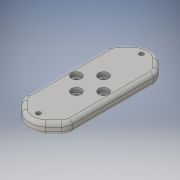
# Autodesk Inventor part: ROV Motor plate
Saved by Autodesk Inventor 2016 (Build 200138000, 138)
## iProperties
Created: 2017-03-09
Part Number: ROV Motor plate
Material: Generic
Document SubType Name: Modeling
Designer: Student
Density: 1 g/cm^3
Appearance: Default
Author: Student
Autodesk Inventor part; units mm, degrees
ref_plane "YZ Plane" through (0, 0, 0) normal (1, 0, 0) x (0, 1, 0)
ref_plane "XZ Plane" through (0, 0, 0) normal (0, 1, 0) x (-1, 0, 0)
ref_plane "XY Plane" through (0, 0, 0) normal (0, 0, 1) x (1, 0, 0)
sketch "Sketch1" plane through (0, 0, 0) normal (0, 1, 0) x (-1, 0, 0)
  line L0 (0, 0) -> (-31.75, 0)
  line L1 (-31.75, 0) -> (-31.75, -77.47)
  line L2 (-31.75, -77.47) -> (0, -77.47)
  line L3 (0, -77.47) -> (0, 0)
  dimension "d0" = 31.75
  dimension "d1" = 77.47
  constraints: 8 end point, 2 parallel, 1 horizontal, 1 perpendicular
  measures "d0" distance of L2.end L1.end
  measures "d1" distance of L1.end L0.end
extrude "Extrusion1" add sketch "Sketch1" along normal blind 7.62
sketch "Sketch2" plane through (0, 7.62, 0) normal (0, 1, 0) x (1, 0, 0)
  line L0 (31.75, 77.47) -> (0, 77.47) projected
  line L1 (0, 0) -> (31.75, 0) projected
  line L2 (0, 77.47) -> (0, 0) projected
  line L3 (31.75, 0) -> (31.75, 77.47) projected
  point P0 (15.875, 74.295)
  point P1 (15.875, 3.175)
  dimension "d6" = 3.175
  dimension "d8" = 15.875
  dimension "d10" = 15.875
  dimension "d37" = 3.175
  measures "d6" distance from line of L1 point (15.875, 3.175)
  measures "d8" distance from line of L2 point (15.875, 3.175)
  measures "d10" distance from line of L2 point (15.875, 74.295)
  measures "d37" distance from line of L0 point (15.875, 74.295)
hole "Hole1" at (15.875, 7.62, -74.295) at (15.875, 7.62, -3.175) direction (0, -1, 0) diameter 3 end through all
sketch "Sketch3" plane through (0, 7.62, 0) normal (0, 1, 0) x (1, 0, 0)
  line L0 (31.75, 0) -> (31.75, 77.47) projected
  line L1 (31.75, 77.47) -> (0, 77.47) projected
  line L2 (15.875, 77.47) -> (15.875, -5.0328) construction
  line L3 (0, 0) -> (31.75, 0) projected
  line L4 (31.75, 38.735) -> (-3.1121, 38.735) construction
  circle A0 centre (15.875, 38.735) radius 9.398
  point P0 (6.477, 38.735)
  point P1 (25.273, 38.735)
  point P2 (15.875, 48.133)
  point P3 (15.875, 29.337)
  constraints: 4 end point, 4 point on line, 3 point on circle, 2 midpoint, 1 centre point, 1 coincident, 1 horizontal, 1 symmetric about line, 1 vertical
hole "Hole2" at (6.477, 7.62, -38.735) at (25.273, 7.62, -38.735) at (15.875, 7.62, -48.133) at (15.875, 7.62, -29.337) direction (0, -1, 0) diameter 3 end through all counterbore diameter 6.87 counterbore depth 2.8
chamfer "Chamfer1" distance 7.62 angle 45 4 edges at (0, 3.81, -77.47) (31.75, 3.81, -77.47) (31.75, 3.81, 0) (0, 3.81, 0)
fillet "Fillet1" radius 7.62 4 edges at (0, 3.81, -69.85) (0, 3.81, -7.62) (31.75, 3.81, -69.85) (31.75, 3.81, -7.62)
sketch "Sketch6" plane through (0, 7.62, 0) normal (0, 1, 0) x (1, 0, 0)
  line L0 (24.13, 77.47) -> (7.62, 77.47) projected
  arc A0 (24.13, 77.47) -> (7.62, 77.47) centre (15.875, 67.8188) ccw
  line L1 (31.75, 10.7763) -> (31.75, 66.6937) projected
  line L2 (31.75, 38.735) -> (-9.2853, 38.735) construction
  line L3 (24.13, 0) -> (7.62, 0)
  arc A1 (7.62, 0) -> (24.13, 0) centre (15.875, 9.6512) ccw
  point P0 (0, 0)
  dimension "d47" = 12.7
  constraints: 4 end point, 4 point on circle, 3 symmetric about line, 2 centre point, 1 horizontal, 1 midpoint, 1 other
  measures "d47" radius of A0
extrude "Extrusion3" add sketch "Sketch6" against normal blind 7.62
fillet "Fillet2" radius 2.54 24 edges at (0.58, 7.62, -7.8603) (4.9259, 7.62, -2.6941) (0.58, 7.62, -69.6097) (4.9259, 7.62, -74.7759) (0, 7.62, -38.735) (0.58, 0, -7.8603) (4.9259, 0, -2.6941) (0.58, 0, -69.6097) (4.9259, 0, -74.7759) (0, 0, -38.735) (31.17, 7.62, -69.6097) (26.8241, 7.62, -74.7759) (31.17, 7.62, -7.8603) (26.8241, 7.62, -2.6941) (31.75, 7.62, -38.735) (31.17, 0, -69.6097) (26.8241, 0, -74.7759) (31.17, 0, -7.8603) (26.8241, 0, -2.6941) (31.75, 0, -38.735) (15.875, 7.62, 3.0488) (15.875, 0, 3.0488) (15.875, 7.62, -80.5188) (15.875, 0, -80.5188)
body "Solid1"
